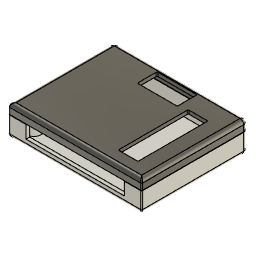
Diag_UP_PCB_v0 v13 (Autodesk Fusion 360 design; units mm, degrees)
Autodesk Fusion 360 part; units mm, degrees
(part 1 of 2)
sketch "Skizze1" plane through (0, 0, 0) normal (0, 0, 1) x (1, 0, 0)
  line L0 (32.8826, 44.1379) -> (33.5317, 44.1379)
  line L1 (32.3975, 53.0162) -> (32.2388, 53.0162)
  line L2 (32.08, 52.8575) -> (32.2388, 53.0162)
  line L3 (31.9213, 53.0162) -> (31.7625, 53.0162)
  line L4 (33.3369, 44.3976) -> (33.3369, 43.8783)
  line L5 (29.286, 48.984) -> (29.286, 48.476)
  line L6 (27.254, 48.476) -> (27.254, 48.984)
  line L7 (31.7625, 53.0162) -> (31.6038, 53.0162)
  line L8 (26.746, 51.016) -> (27.254, 51.016)
  line L9 (29.794, 48.476) -> (29.794, 48.984)
  line L10 (33.1422, 45.0467) -> (32.8826, 44.1379)
  line L11 (27.254, 48.984) -> (26.746, 48.984)
  line L12 (27.254, 51.524) -> (26.746, 51.524)
  line L13 (29.794, 48.984) -> (29.286, 48.984)
  arc A0 (34.62, 45.3962) -> (35.89, 45.3962) centre (35.255, 45.3962) ccw
  line L14 (32.334, 48.476) -> (32.334, 48.984)
  line L15 (32.715, 53.0162) -> (32.5563, 53.0162)
  line L16 (31.445, 53.0162) -> (32.08, 52.3812)
  line L17 (36.3663, 46.19) -> (35.89, 46.6662)
  line L18 (32.08, 52.6987) -> (32.3975, 53.0162)
  line L19 (31.6038, 53.0162) -> (31.445, 53.0162)
  line L20 (24.206, 51.016) -> (24.714, 51.016)
  line L21 (22.174, 51.016) -> (22.174, 51.524)
  line L22 (24.714, 48.984) -> (24.206, 48.984)
  line L23 (22.174, 48.984) -> (21.666, 48.984)
  line L24 (24.714, 48.476) -> (24.714, 48.984)
  line L25 (29.794, 51.016) -> (29.794, 51.524)
  arc A1 (18.11, 45.3962) -> (19.38, 45.3962) centre (18.745, 45.3962) ccw
  line L26 (36.3663, 53.81) -> (35.89, 53.3338)
  line L27 (31.826, 48.476) -> (32.334, 48.476)
  line L28 (24.206, 48.476) -> (24.714, 48.476)
  line L29 (26.746, 48.476) -> (27.254, 48.476)
  line L30 (21.666, 51.016) -> (22.174, 51.016)
  line L31 (32.334, 51.016) -> (32.334, 51.524)
  line L32 (27.254, 51.016) -> (27.254, 51.524)
  line L33 (31.826, 48.984) -> (31.826, 48.476)
  line L34 (21.666, 48.476) -> (22.174, 48.476)
  line L35 (31.826, 51.524) -> (31.826, 51.016)
  line L36 (26.746, 48.984) -> (26.746, 48.476)
  line L37 (21.666, 51.524) -> (21.666, 51.016)
  line L38 (29.286, 51.524) -> (29.286, 51.016)
  arc A2 (26.5238, 45.3962) -> (27.635, 45.3962) centre (27.0794, 45.3962) ccw
  line L39 (21.666, 48.984) -> (21.666, 48.476)
  line L40 (32.0956, 43.8783) -> (31.9657, 43.8783)
  line L41 (24.206, 48.984) -> (24.206, 48.476)
  line L42 (32.08, 52.3812) -> (32.715, 53.0162)
  line L43 (29.0638, 53.81) -> (36.3663, 53.81)
  line L44 (22.174, 51.524) -> (21.666, 51.524)
  arc A3 (32.0956, 43.8783) -> (32.3552, 44.1379) centre (32.0956, 44.1379) ccw
  line L45 (24.714, 51.016) -> (24.714, 51.524)
  line L46 (32.5563, 53.0162) -> (32.3975, 53.0162)
  line L47 (32.08, 52.54) -> (32.5563, 53.0162)
  line L48 (29.794, 51.524) -> (29.286, 51.524)
  line L49 (18.11, 53.3338) -> (17.6337, 53.81)
  line L50 (17.6337, 48.2537) -> (17.6337, 53.81)
  line L51 (29.286, 51.016) -> (29.794, 51.016)
  line L52 (32.334, 48.984) -> (31.826, 48.984)
  line L53 (24.206, 51.524) -> (24.206, 51.016)
  line L54 (26.746, 51.524) -> (26.746, 51.016)
  line L55 (22.174, 48.476) -> (22.174, 48.984)
  line L56 (24.714, 51.524) -> (24.206, 51.524)
  line L57 (32.3552, 45.0467) -> (32.3552, 44.1379)
  line L58 (29.286, 48.476) -> (29.794, 48.476)
  line L59 (35.4013, 18.415) -> (35.4013, 17.653)
  line L60 (40.0695, 44.5417) -> (40.3941, 44.5417)
  line L61 (39.37, 33.4963) -> (39.37, 41.1163)
  line L62 (39.6875, 41.1163) -> (39.6875, 33.4963)
  line L63 (40.0695, 43.3733) -> (40.0695, 44.5417)
  line L64 (41.5297, 44.5417) -> (41.5297, 43.3733)
  line L65 (36.83, 41.1163) -> (36.83, 33.4963)
  line L66 (41.2052, 44.2821) -> (41.5297, 44.5417)
  line L67 (40.9575, 41.1163) -> (40.9575, 41.8783)
  line L68 (42.2275, 41.1163) -> (39.6875, 41.1163)
  line L69 (36.6713, 18.415) -> (36.6713, 26.035)
  arc A4 (38.7569, 44.1649) -> (38.8543, 44.3921) centre (38.5405, 44.3921) ccw
  line L70 (40.3941, 43.8926) -> (40.0695, 43.8926)
  line L71 (34.1313, 26.035) -> (34.1313, 18.415)
  arc A5 (38.8543, 44.3921) -> (38.5622, 44.6842) centre (38.5622, 44.3921) ccw
  line L72 (37.3941, 44.0351) -> (37.0695, 44.0351)
  line L73 (39.37, 41.1163) -> (36.83, 41.1163)
  line L74 (38.1, 41.1163) -> (38.1, 41.8783)
  line L75 (36.83, 33.4963) -> (39.37, 33.4963)
  line L76 (37.0695, 44.6842) -> (37.3941, 44.6842)
  line L77 (40.9575, 33.4963) -> (40.9575, 32.7343)
  line L78 (39.6875, 33.4963) -> (42.2275, 33.4963)
  line L79 (37.0695, 43.5158) -> (37.0695, 44.6842)
  line L80 (37.7187, 43.5158) -> (37.459, 44.0351)
  line L81 (40.7187, 43.3733) -> (40.459, 43.8926)
  line L82 (42.2275, 33.4963) -> (42.2275, 41.1163)
  arc A6 (40.3941, 43.8925) -> (40.3941, 44.5417) centre (40.3941, 44.2171) ccw
  line L83 (38.2052, 43.5158) -> (38.8543, 43.5158)
  arc A7 (37.3941, 44.035) -> (37.3941, 44.6842) centre (37.3941, 44.3596) ccw
  line L84 (38.7569, 44.1649) -> (38.2052, 43.5158)
  line L85 (38.1, 33.4963) -> (38.1, 32.7343)
  line L86 (41.2052, 43.3733) -> (41.8543, 43.3733)
  arc A8 (38.5622, 44.6842) -> (38.2052, 44.4245) centre (38.5622, 44.3089) ccw
  line L87 (5.89, 0.1) -> (5.89, -1)
  line L88 (30.38, 0) -> (30.38, -1)
  line L89 (13.31, 3) -> (13.31, 2)
  line L90 (13.81, 0.1) -> (13.81, 4)
  line L91 (16.27, 3) -> (16.27, 2)
  arc A9 (28.15, 2) -> (29.15, 2) centre (28.65, 2) ccw
  arc A10 (17.27, 3) -> (16.27, 3) centre (16.77, 3) ccw
  line L92 (19, -1) -> (19, 0)
  line L93 (26.92, 0) -> (26.42, 0)
  line L94 (17.77, 0.1) -> (17.77, -1)
  line L95 (15.04, -1) -> (15.04, 0)
  line L96 (17.77, 0.1) -> (17.77, 4)
  line L97 (24.19, 3) -> (24.19, 2)
  line L98 (13.81, 0.1) -> (13.81, -1)
  arc A11 (13.31, 3) -> (12.31, 3) centre (12.81, 3) ccw
  line L99 (17.27, 3) -> (17.27, 2)
  line L100 (11.08, -1) -> (11.08, 0)
  line L101 (21.73, 0.1) -> (21.73, -1)
  line L102 (23.69, 0.1) -> (23.69, -1)
  arc A12 (17.77, 4) -> (15.77, 4) centre (16.77, 4) ccw
  line L103 (21.73, 0.1) -> (21.73, 4)
  line L104 (14.54, 0) -> (14.54, -1)
  line L105 (11.08, 0) -> (10.58, 0)
  line L106 (12.31, 3) -> (12.31, 2)
  arc A13 (13.81, 4) -> (11.81, 4) centre (12.81, 4) ccw
  arc A14 (16.27, 2) -> (17.27, 2) centre (16.77, 2) ccw
  line L107 (6.62, 0) -> (6.62, -1)
  line L108 (30.88, 0) -> (30.38, 0)
  line L109 (21.23, 3) -> (21.23, 2)
  line L110 (3.89, 0.1) -> (3.89, 4)
  arc A15 (24.19, 2) -> (25.19, 2) centre (24.69, 2) ccw
  line L111 (18.5, 0) -> (18.5, -1)
  arc A16 (25.69, 4) -> (23.69, 4) centre (24.69, 4) ccw
  line L112 (29.65, 0.1) -> (29.65, 4)
  arc A17 (21.73, 4) -> (19.73, 4) centre (20.73, 4) ccw
  line L113 (11.81, 0.1) -> (11.81, 4)
  line L114 (20.23, 3) -> (20.23, 2)
  line L115 (15.04, 0) -> (14.54, 0)
  arc A18 (12.31, 2) -> (13.31, 2) centre (12.81, 2) ccw
  arc A19 (9.35, 3) -> (8.35, 3) centre (8.85, 3) ccw
  line L116 (15.77, 0.1) -> (15.77, -1)
  line L117 (19.73, 0.1) -> (19.73, -1)
  line L118 (9.85, 0.1) -> (9.85, 4)
  arc A20 (8.35, 2) -> (9.35, 2) centre (8.85, 2) ccw
  line L119 (7.12, 0) -> (6.62, 0)
  line L120 (11.81, 0.1) -> (11.81, -1)
  line L121 (19.73, 0.1) -> (19.73, 4)
  arc A21 (21.23, 3) -> (20.23, 3) centre (20.73, 3) ccw
  line L122 (10.58, 0) -> (10.58, -1)
  arc A22 (20.23, 2) -> (21.23, 2) centre (20.73, 2) ccw
  line L123 (19, 0) -> (18.5, 0)
  line L124 (2.66, 0) -> (2.66, -1)
  line L125 (4.39, 3) -> (4.39, 2)
  line L126 (7.12, -1) -> (7.12, 0)
  line L127 (5.89, 0.1) -> (5.89, 4)
  line L128 (15.77, 0.1) -> (15.77, 4)
  line L129 (28.15, 3) -> (28.15, 2)
  line L130 (22.46, 0) -> (22.46, -1)
  arc A23 (9.85, 4) -> (7.85, 4) centre (8.85, 4) ccw
  arc A24 (5.89, 4) -> (3.89, 4) centre (4.89, 4) ccw
  line L131 (8.35, 3) -> (8.35, 2)
  line L132 (-6.03, 0) -> (-7.58, 0)
  line L133 (-0.13, -1) -> (-0.13, 0)
  line L134 (-6.03, -1.6) -> (-6.03, 0)
  line L135 (59.37, -6.8) -> (55.97, -6.8)
  line L136 (59.37, 0) -> (57.67, 0)
  line L137 (7.85, 0.1) -> (7.85, 4)
  line L138 (-6.03, -6.8) -> (-6.03, -5.2)
  line L139 (60.92, -6.8) -> (59.37, -6.8)
  line L140 (3.89, 0.1) -> (3.89, -1)
  line L141 (5.39, 3) -> (5.39, 2)
  line L142 (59.37, -6.8) -> (59.37, -5.2)
  line L143 (3.16, -1) -> (3.16, 0)
  line L144 (57.67, -2.8667) -> (57.67, 0)
  line L145 (57.67, -3.6853) -> (57.67, -3.548)
  line L146 (-4.33, 0) -> (-6.03, 0)
  line L147 (-4.33, -4.3667) -> (-4.33, -7.2333)
  line L148 (57.67, 0) -> (55.97, 0)
  line L149 (-0.83, -6.8) -> (-2.63, -6.8)
  arc A25 (4.39, 2) -> (5.39, 2) centre (4.89, 2) ccw
  line L150 (-4.33, -8.7333) -> (-4.33, -11.6)
  line L151 (7.85, 0.1) -> (7.85, -1)
  line L152 (-0.83, -11.6) -> (-0.83, -6.8)
  line L153 (55.97, -6.8) -> (54.17, -6.8)
  line L154 (53.47, -1) -> (-0.13, -1)
  line L155 (-6.03, -4.2) -> (-6.03, -2.6)
  line L156 (3.16, 0) -> (2.66, 0)
  line L157 (9.85, 0.1) -> (9.85, -1)
  line L158 (59.37, -4.2) -> (59.37, -2.6)
  line L159 (-2.63, -6.8) -> (-2.63, -5.2)
  line L160 (57.67, -7.2333) -> (57.67, -4.3667)
  line L161 (9.35, 3) -> (9.35, 2)
  line L162 (-4.33, -7.9147) -> (-4.33, -8.052)
  line L163 (55.97, 0) -> (53.47, 0)
  line L164 (-0.13, 0) -> (-2.63, 0)
  line L165 (53.47, 0) -> (53.47, -1)
  line L166 (-2.63, 0) -> (-4.33, 0)
  line L167 (60.92, 0) -> (59.37, 0)
  line L168 (-2.63, -6.8) -> (-6.03, -6.8)
  line L169 (60.92, 0) -> (60.92, -6.8)
  line L170 (57.67, -8.052) -> (57.67, -7.9147)
  line L171 (-2.63, -4.2) -> (-2.63, -2.6)
  arc A26 (5.39, 3) -> (4.39, 3) centre (4.89, 3) ccw
  line L172 (-7.58, 0) -> (-7.58, -6.8)
  line L173 (-4.33, -3.548) -> (-4.33, -3.6853)
  line L174 (52.6038, 8.38) -> (46.2537, 8.38)
  line L175 (51.5814, 0.7496) -> (52.2305, 0.7496)
  line L176 (51.3338, 9.65) -> (46.2537, 9.65)
  line L177 (54.17, -11.6) -> (-0.83, -11.6)
  line L178 (46.2537, 9.65) -> (44.825, 9.65)
  line L179 (44.825, 9.65) -> (44.6662, 9.65)
  line L180 (51.5814, 1.6583) -> (51.9059, 1.918)
  line L181 (51.3338, 14.73) -> (51.3338, 9.65)
  line L182 (51.3338, 14.73) -> (51.81, 14.73)
  line L183 (51.9059, 1.918) -> (51.9059, 0.7496)
  line L184 (51.054, 1.918) -> (51.054, 1.0092)
  line L185 (46.2537, 23.62) -> (52.6038, 23.62)
  line L186 (44.825, 8.38) -> (43.3962, 8.38)
  line L187 (44.825, 22.35) -> (46.2537, 22.35)
  line L188 (43.3962, 23.62) -> (44.825, 23.62)
  line L189 (-6.03, -6.8) -> (-7.58, -6.8)
  line L190 (54.17, -6.8) -> (54.17, -11.6)
  line L191 (50.7944, 0.7496) -> (50.6646, 0.7496)
  line L192 (51.3338, 17.27) -> (51.3338, 14.73)
  line L193 (-4.33, 0) -> (-4.33, -2.8667)
  line L194 (57.67, -11.6) -> (57.67, -8.7333)
  line L195 (-2.63, -1.6) -> (-2.63, 0)
  line L196 (51.3338, 22.35) -> (51.3338, 17.27)
  line L197 (51.81, 14.73) -> (52.6038, 14.73)
  line L198 (51.81, 9.1737) -> (51.3338, 9.65)
  line L199 (51.0162, 13.7775) -> (51.0162, 13.9362)
  line L200 (46.2537, 22.8263) -> (51.81, 22.8263)
  line L201 (46.2537, 22.8263) -> (46.2537, 23.62)
  line L202 (46.2537, 9.1737) -> (51.81, 9.1737)
  line L203 (46.2537, 22.35) -> (51.3338, 22.35)
  line L204 (44.19, 9.1737) -> (44.6662, 9.65)
  line L205 (55.97, -4.2) -> (55.97, -2.6)
  line L206 (52.6038, 23.62) -> (52.6038, 17.27)
  line L207 (52.6038, 14.73) -> (52.6038, 8.38)
  arc A27 (50.7944, 0.7496) -> (51.054, 1.0092) centre (50.7944, 1.0092) ccw
  line L208 (50.54, 13.46) -> (51.0162, 12.9837)
  line L209 (46.2537, 22.35) -> (46.2537, 22.8263)
  line L210 (44.825, 22.8263) -> (44.19, 22.8263)
  line L211 (55.97, -6.8) -> (55.97, -5.2)
  line L212 (44.825, 9.65) -> (44.825, 9.1737)
  line L213 (51.3338, 17.27) -> (51.81, 17.27)
  line L214 (50.3812, 13.46) -> (51.0162, 12.825)
  line L215 (51.81, 17.27) -> (51.81, 22.8263)
  line L216 (44.6662, 22.35) -> (44.19, 22.8263)
  line L217 (46.2537, 9.1737) -> (46.2537, 8.38)
  line L218 (44.825, 22.35) -> (44.825, 22.8263)
  line L219 (51.81, 14.73) -> (51.81, 9.1737)
  arc A28 (43.3962, 16.4763) -> (43.3962, 15.3651) centre (43.3962, 15.9207) ccw
  line L220 (51.0162, 13.9362) -> (51.0162, 14.095)
  line L221 (46.2537, 8.38) -> (44.825, 8.38)
  line L222 (44.6662, 9.65) -> (44.6662, 22.35)
  line L223 (52.6038, 17.27) -> (52.6038, 14.73)
  line L224 (44.19, 9.1737) -> (44.19, 22.8263)
  line L225 (51.81, 17.27) -> (52.6038, 17.27)
  line L226 (44.825, 9.1737) -> (44.825, 8.38)
  line L227 (44.825, 22.8263) -> (44.825, 23.62)
  line L228 (59.37, -1.6) -> (59.37, 0)
  line L229 (43.3962, 8.38) -> (43.3962, 23.62)
  line L230 (44.6662, 22.35) -> (44.825, 22.35)
  line L231 (44.19, 9.1737) -> (44.825, 9.1737)
  arc A29 (43.3962, 10.92) -> (43.3962, 9.65) centre (43.3962, 10.285) ccw
  line L232 (51.0162, 12.825) -> (51.0162, 12.9837)
  line L233 (51.0162, 14.095) -> (50.3812, 13.46)
  line L234 (46.2537, 9.65) -> (46.2537, 9.1737)
  line L235 (44.825, 23.62) -> (46.2537, 23.62)
  line L236 (51.3338, 22.35) -> (51.81, 22.8263)
  arc A30 (43.3962, 22.35) -> (43.3962, 21.08) centre (43.3962, 21.715) ccw
  line L237 (51.0162, 13.9362) -> (50.54, 13.46)
  line L238 (55.97, -1.6) -> (55.97, 0)
  line L239 (43.3962, 24.84) -> (43.3962, 45.16)
  line L240 (52.6038, 32.9362) -> (52.6038, 24.84)
  line L241 (44.825, 25.6337) -> (44.825, 24.84)
  line L242 (49.524, 13.206) -> (49.524, 13.714)
  line L243 (46.2537, 26.11) -> (46.2537, 25.6337)
  line L244 (46.2537, 43.89) -> (51.3338, 43.89)
  line L245 (42.6867, 14.7564) -> (42.6867, 15.4055)
  line L246 (49.016, 18.794) -> (49.016, 18.286)
  line L247 (51.3338, 43.89) -> (51.3338, 37.0638)
  line L248 (49.524, 15.746) -> (49.524, 16.254)
  line L249 (46.984, 15.746) -> (46.984, 16.254)
  line L250 (46.476, 18.794) -> (46.476, 18.286)
  line L251 (49.524, 13.714) -> (49.016, 13.714)
  line L252 (46.2537, 45.16) -> (52.6038, 45.16)
  line L253 (46.984, 13.206) -> (46.984, 13.714)
  line L254 (51.0162, 13.6187) -> (50.8575, 13.46)
  arc A31 (41.5183, 15.1134) -> (41.778, 14.7564) centre (41.8936, 15.1134) ccw
  line L255 (51.0162, 13.3012) -> (51.0162, 13.6187)
  line L256 (49.016, 18.286) -> (49.524, 18.286)
  line L257 (42.6867, 13.9694) -> (42.6867, 13.8396)
  line L258 (46.984, 18.794) -> (46.476, 18.794)
  line L259 (46.476, 13.714) -> (46.476, 13.206)
  line L260 (46.476, 15.746) -> (46.984, 15.746)
  line L261 (49.524, 18.794) -> (49.016, 18.794)
  arc A32 (42.6867, 13.9694) -> (42.4271, 14.229) centre (42.4271, 13.9694) ccw
  line L262 (46.2537, 26.11) -> (44.825, 26.11)
  line L263 (49.524, 16.254) -> (49.016, 16.254)
  arc A33 (41.8104, 15.4055) -> (41.5183, 15.1134) centre (41.8104, 15.1134) ccw
  line L264 (51.3338, 37.0638) -> (51.81, 37.0638)
  line L265 (44.825, 45.16) -> (46.2537, 45.16)
  line L266 (49.016, 13.206) -> (49.524, 13.206)
  line L267 (46.984, 13.714) -> (46.476, 13.714)
  line L268 (46.984, 18.286) -> (46.984, 18.794)
  line L269 (52.6038, 37.0638) -> (52.6038, 32.9362)
  line L270 (44.825, 44.3663) -> (44.825, 45.16)
  line L271 (44.825, 26.11) -> (44.825, 25.6337)
  line L272 (44.6662, 26.11) -> (44.6662, 43.89)
  line L273 (50.6987, 13.46) -> (51.0162, 13.1425)
  line L274 (46.476, 16.254) -> (46.476, 15.746)
  line L275 (49.016, 15.746) -> (49.524, 15.746)
  arc A34 (42.0376, 15.3081) -> (41.8104, 15.4055) centre (41.8104, 15.0918) ccw
  line L276 (41.5183, 14.2291) -> (42.4271, 14.2291)
  line L277 (51.0162, 13.1425) -> (51.0162, 13.3012)
  line L278 (46.984, 16.254) -> (46.476, 16.254)
  line L279 (51.0162, 12.9837) -> (51.0162, 13.1425)
  line L280 (51.0162, 13.7775) -> (50.6987, 13.46)
  line L281 (46.476, 18.286) -> (46.984, 18.286)
  line L282 (50.8575, 13.46) -> (51.0162, 13.3012)
  line L283 (49.524, 18.286) -> (49.524, 18.794)
  line L284 (46.476, 13.206) -> (46.984, 13.206)
  line L285 (49.016, 13.714) -> (49.016, 13.206)
  line L286 (51.3338, 26.11) -> (46.2537, 26.11)
  line L287 (49.016, 16.254) -> (49.016, 15.746)
  line L288 (44.825, 43.89) -> (44.825, 44.3663)
  line L289 (51.0162, 13.6187) -> (51.0162, 13.7775)
  line L290 (51.81, 32.9362) -> (51.81, 25.6337)
  line L291 (51.0162, 30.0787) -> (50.8575, 29.92)
  line L292 (51.0162, 30.3962) -> (50.54, 29.92)
  line L293 (51.81, 32.9362) -> (52.6038, 32.9362)
  line L294 (45.3675, 6.9448) -> (44.8708, 7.2157)
  line L295 (46.984, 32.206) -> (46.984, 32.714)
  line L296 (44.825, 44.3663) -> (44.19, 44.3663)
  line L297 (51.3338, 32.9362) -> (51.81, 32.9362)
  line L298 (51.3338, 37.0638) -> (51.3338, 32.9362)
  line L299 (51.0162, 29.6025) -> (51.0162, 29.7612)
  line L300 (44.6662, 43.89) -> (44.825, 43.89)
  line L301 (46.2537, 43.89) -> (46.2537, 44.3663)
  line L302 (52.4567, 6.2675) -> (51.7342, 6.2675)
  line L303 (45.411, 47.263) -> (46.3142, 47.263)
  line L304 (44.19, 25.6337) -> (44.825, 25.6337)
  line L305 (46.9312, 45.6375) -> (46.9312, 47.263)
  line L306 (51.0162, 29.285) -> (51.0162, 29.4437)
  line L307 (44.6662, 43.89) -> (44.19, 44.3663)
  line L308 (44.825, 26.11) -> (44.6662, 26.11)
  line L309 (52.6038, 24.84) -> (46.2537, 24.84)
  line L310 (51.0162, 30.0787) -> (51.0162, 30.2375)
  arc A35 (43.3962, 27.38) -> (43.3962, 26.11) centre (43.3962, 26.745) ccw
  arc A36 (46.9167, 7.7575) -> (46.5103, 7.893) centre (46.5103, 7.2157) ccw
  line L311 (51.81, 37.0638) -> (52.6038, 37.0638)
  line L312 (51.81, 25.6337) -> (51.3338, 26.11)
  line L313 (46.2537, 25.6337) -> (51.81, 25.6337)
  line L314 (50.3812, 29.92) -> (51.0162, 29.285)
  line L315 (46.2537, 24.84) -> (44.825, 24.84)
  line L316 (52.6038, 45.16) -> (52.6038, 37.0638)
  line L317 (51.0162, 30.555) -> (50.3812, 29.92)
  line L318 (50.54, 29.92) -> (51.0162, 29.4437)
  line L319 (51.0162, 30.2375) -> (51.0162, 30.3962)
  line L320 (50.6987, 29.92) -> (51.0162, 29.6025)
  arc A37 (47.0071, 6.6287) -> (46.8265, 6.9448) centre (46.6402, 6.6287) ccw
  line L321 (44.19, 25.6337) -> (44.6662, 26.11)
  line L322 (46.2537, 44.3663) -> (51.81, 44.3663)
  arc A38 (43.3962, 35.4763) -> (43.3962, 34.3651) centre (43.3962, 34.9207) ccw
  arc A39 (45.0514, 7.893) -> (44.6902, 7.5318) centre (45.0514, 7.5318) ccw
  line L323 (43.3962, 45.16) -> (44.825, 45.16)
  line L324 (51.0162, 29.4437) -> (51.0162, 29.6025)
  line L325 (46.2537, 25.6337) -> (46.2537, 24.84)
  line L326 (51.0162, 30.3962) -> (51.0162, 30.555)
  line L327 (51.7342, 6.2675) -> (51.7342, 7.8931)
  arc A40 (45.4578, 7.7575) -> (45.0514, 7.893) centre (45.0514, 7.2157) ccw
  arc A41 (46.104, 6.4933) -> (46.6458, 6.2675) centre (46.6458, 7.0306) ccw
  line L328 (49.317, 6.2675) -> (49.317, 7.8931)
  line L329 (42.0376, 15.3081) -> (42.6867, 14.7564)
  line L330 (51.3338, 32.9362) -> (51.3338, 26.11)
  line L331 (50.8575, 29.92) -> (51.0162, 29.7612)
  line L332 (51.0162, 29.7612) -> (51.0162, 30.0787)
  line L333 (45.8626, 45.6375) -> (45.8626, 47.263)
  line L334 (44.825, 43.89) -> (46.2537, 43.89)
  arc A42 (43.3962, 43.89) -> (43.3962, 42.62) centre (43.3962, 43.255) ccw
  line L335 (47.67, 7.8931) -> (48.3925, 7.8931)
  line L336 (44.825, 24.84) -> (43.3962, 24.84)
  line L337 (50.6717, 6.2675) -> (50.6717, 7.8931)
  line L338 (46.2537, 44.3663) -> (46.2537, 45.16)
  line L339 (51.81, 37.0638) -> (51.81, 44.3663)
  line L340 (50.2202, 7.8931) -> (51.1233, 7.8931)
  line L341 (51.0162, 30.2375) -> (50.6987, 29.92)
  line L342 (51.3338, 43.89) -> (51.81, 44.3663)
  line L343 (44.19, 25.6337) -> (44.19, 44.3663)
  arc A43 (45.5481, 6.6287) -> (45.3675, 6.9448) centre (45.1812, 6.6287) ccw
  line L344 (48.3925, 6.2675) -> (47.67, 6.2675)
  arc A44 (46.6458, 6.2675) -> (47.007, 6.6287) centre (46.6458, 6.6287) ccw
  line L345 (37.827, 47.1573) -> (37.827, 48.0604)
  line L346 (48.8655, 7.8931) -> (49.7686, 7.8931)
  arc A45 (44.6902, 7.5318) -> (44.8708, 7.2157) centre (45.0571, 7.5318) ccw
  arc A46 (5.1626, 14.8153) -> (4.711, 15.2669) centre (4.711, 14.8153) ccw
  line L347 (0, 1) -> (0, 54)
  line L348 (3.9885, 15.2668) -> (4.711, 15.2668)
  arc A47 (47.3828, 46.3599) -> (47.3828, 47.2631) centre (47.3828, 46.8115) ccw
  line L349 (44.2087, 45.9987) -> (44.2087, 46.9018)
  line L350 (47.8343, 45.6375) -> (47.4731, 46.3599)
  line L351 (49.8017, 46.7212) -> (50.8854, 46.7212)
  arc A48 (52, 0) -> (53, 1) centre (52, 1) ccw
  arc A49 (0, 1) -> (1, 0) centre (1, 1) ccw
  line L352 (47.67, 7.1706) -> (48.2119, 7.1706)
  arc A50 (44.2087, 45.9987) -> (44.5699, 45.6375) centre (44.5699, 45.9987) ccw
  line L353 (47.67, 6.2675) -> (47.67, 7.8931)
  line L354 (39.4526, 46.6774) -> (39.4526, 46.3162)
  arc A51 (39.0913, 45.955) -> (39.4525, 46.3162) centre (39.0913, 46.3162) ccw
  line L355 (46.9312, 47.263) -> (47.3828, 47.263)
  arc A52 (53, 54) -> (52, 55) centre (52, 54) ccw
  line L356 (39.4526, 48.6775) -> (37.827, 48.6775)
  arc A53 (1, 55) -> (0, 54) centre (1, 54) ccw
  line L357 (3.537, 14.3637) -> (3.537, 14.8153)
  arc A54 (4.6207, 21.1545) -> (4.2595, 20.7933) centre (4.6207, 20.7933) ccw
  line L358 (48.5403, 45.6375) -> (49.2628, 45.6375)
  line L359 (37.827, 46.3162) -> (37.827, 46.6774)
  line L360 (50.6145, 45.6375) -> (50.6145, 47.263)
  line L361 (53, 1) -> (53, 54)
  line L362 (4.5304, 17.3054) -> (4.5304, 16.899)
  line L363 (46.8264, 6.9448) -> (46.3297, 7.2157)
  arc A55 (37.8269, 46.3162) -> (38.1882, 45.9549) centre (38.1882, 46.3162) ccw
  arc A56 (46.5103, 7.893) -> (46.1491, 7.5318) centre (46.5103, 7.5318) ccw
  arc A57 (44.5699, 47.263) -> (44.2087, 46.9018) centre (44.5699, 46.9018) ccw
  arc A58 (46.1491, 7.5318) -> (46.3297, 7.2157) centre (46.516, 7.5318) ccw
  line L364 (48.5403, 47.263) -> (48.5403, 45.6375)
  line L365 (51.7342, 7.8931) -> (52.4567, 7.8931)
  line L366 (44.5699, 47.263) -> (44.9312, 47.263)
  line L367 (51.5072, 46.9018) -> (51.9588, 47.263)
  line L368 (51.9588, 47.263) -> (51.9588, 45.6375)
  line L369 (50.0726, 45.6375) -> (50.0726, 47.263)
  line L370 (39.4526, 47.6088) -> (37.827, 47.6088)
  line L371 (51.5072, 45.6375) -> (52.4103, 45.6375)
  line L372 (51.7342, 7.1706) -> (52.276, 7.1706)
  line L373 (44.9312, 45.6375) -> (44.5699, 45.6375)
  line L374 (47.3828, 46.3599) -> (46.9312, 46.3599)
  line L375 (1, 0) -> (52, 0)
  line L376 (5.1626, 14.3637) -> (3.537, 14.3637)
  line L377 (49.8017, 46.1793) -> (50.8854, 46.1793)
  line L378 (39.0913, 45.955) -> (38.1882, 45.955)
  arc A59 (3.9885, 15.2669) -> (3.5369, 14.8153) centre (3.9885, 14.8153) ccw
  line L379 (52, 55) -> (1, 55)
  line L380 (4.0788, 17.0345) -> (4.0788, 16.6733)
  line L381 (4.2594, 20.7933) -> (4.2594, 20.2515)
  line L382 (4.2594, 20.2515) -> (3.537, 20.2515)
  line L383 (4.711, 32.7043) -> (4.5304, 32.2528)
  arc A60 (4.711, 30.5159) -> (4.711, 31.4191) centre (4.711, 30.9675) ccw
  line L384 (4.0788, 18.2607) -> (4.0788, 18.7122)
  arc A61 (4.3498, 17.3054) -> (4.0789, 17.0345) centre (4.3498, 17.0345) ccw
  arc A62 (4.5304, 16.899) -> (5.1626, 16.899) centre (4.8465, 16.899) ccw
  line L385 (4.711, 31.4191) -> (3.537, 31.4191)
  arc A63 (3.7628, 28.2026) -> (4.3498, 28.0671) centre (4.3498, 29.4067) ccw
  line L386 (5.1626, 16.899) -> (5.1626, 17.3054)
  arc A64 (4.3498, 28.9701) -> (3.7628, 28.8346) centre (4.3498, 27.6305) ccw
  line L387 (5.1626, 17.3054) -> (4.3498, 17.3054)
  arc A65 (4.0789, 18.2607) -> (4.3498, 17.9898) centre (4.3498, 18.2607) ccw
  arc A66 (5.0722, 32.1173) -> (5.1625, 32.614) centre (3.6311, 32.6359) ccw
  line L388 (3.6273, 15.9164) -> (3.537, 15.9164)
  line L389 (3.537, 15.9164) -> (3.537, 16.0067)
  arc A67 (3.537, 27.0007) -> (3.8982, 26.504) centre (4.0591, 27.0007) ccw
  arc A68 (3.8982, 21.9049) -> (3.8982, 22.6273) centre (3.8982, 22.2661) ccw
  line L390 (4.2594, 25.7085) -> (5.1626, 24.9408)
  arc A69 (4.9368, 28.8346) -> (4.3498, 28.9701) centre (4.3498, 27.6305) ccw
  line L391 (5.1626, 15.9615) -> (4.0788, 15.9615)
  arc A70 (4.711, 21.8145) -> (4.711, 22.7177) centre (4.711, 22.2661) ccw
  line L392 (4.8013, 21.1546) -> (4.6207, 21.1546)
  arc A71 (4.711, 23.3777) -> (4.711, 24.2809) centre (4.711, 23.8293) ccw
  line L393 (5.1626, 20.2515) -> (5.1626, 20.7933)
  arc A72 (3.537, 25.4375) -> (3.8982, 24.9408) centre (4.0591, 25.4375) ccw
  arc A73 (4.2595, 27.2715) -> (3.9434, 27.407) centre (3.9434, 26.9705) ccw
  line L394 (3.537, 20.2515) -> (3.537, 21.1546)
  line L395 (3.537, 16.0067) -> (3.6273, 16.0067)
  arc A74 (4.8916, 17.9898) -> (5.1625, 18.2607) centre (4.8916, 18.2607) ccw
  line L396 (4.8916, 17.9898) -> (4.3498, 17.9898)
  arc A75 (4.711, 22.7177) -> (4.711, 21.8145) centre (4.711, 22.2661) ccw
  arc A76 (4.6207, 24.2808) -> (4.2595, 23.9196) centre (4.6207, 23.9196) ccw
  line L397 (4.2594, 23.3777) -> (4.2594, 23.9196)
  arc A77 (3.9434, 25.8439) -> (3.537, 25.4375) centre (3.9434, 25.4375) ccw
  line L398 (4.2594, 27.2716) -> (5.1626, 26.5039)
  arc A78 (5.1625, 20.7933) -> (4.8013, 21.1545) centre (4.8013, 20.7933) ccw
  arc A79 (5.7044, 18.4413) -> (5.4335, 18.7122) centre (5.4335, 18.4413) ccw
  arc A80 (3.5369, 24.1002) -> (4.2594, 23.3777) centre (4.2594, 24.1002) ccw
  arc A81 (3.7627, 28.8347) -> (3.5369, 28.5186) centre (3.8711, 28.5186) ccw
  arc A82 (4.9368, 28.2025) -> (5.1626, 28.5186) centre (4.8284, 28.5186) ccw
  arc A83 (4.0788, 32.343) -> (4.5304, 32.2527) centre (4.313, 32.3397) ccw
  arc A84 (3.9434, 27.4071) -> (3.537, 27.0007) centre (3.9434, 27.0007) ccw
  arc A85 (5.1626, 32.614) -> (4.711, 32.7043) centre (4.9284, 32.6173) ccw
  line L399 (4.0788, 18.7122) -> (5.4335, 18.7122)
  arc A86 (4.1691, 32.7495) -> (4.0788, 32.343) centre (5.1043, 32.3284) ccw
  arc A87 (3.8982, 22.6273) -> (3.8982, 21.9049) centre (3.8982, 22.2661) ccw
  arc A88 (4.2595, 25.7084) -> (3.9434, 25.8439) centre (3.9434, 25.4074) ccw
  line L400 (5.1626, 18.7122) -> (5.1626, 18.2607)
  line L401 (5.7044, 18.4413) -> (5.7044, 18.0801)
  line L402 (4.6207, 24.2808) -> (4.711, 24.2808)
  line L403 (4.8013, 28.1574) -> (3.8982, 28.8799)
  line L404 (5.1626, 14.8153) -> (5.1626, 14.3637)
  line L405 (3.6273, 16.0067) -> (3.6273, 15.9164)
  line L406 (5.1626, 26.5039) -> (5.1626, 27.4071)
  line L407 (4.711, 23.3777) -> (4.2594, 23.3777)
  line L408 (50.68, -1) -> (50.68, 0)
  line L409 (38.8, 0) -> (38.3, 0)
  line L410 (46.72, 0) -> (46.22, 0)
  line L411 (47.45, 0.1) -> (47.45, -1)
  line L412 (32.11, 3) -> (32.11, 2)
  arc A89 (33.11, 3) -> (32.11, 3) centre (32.61, 3) ccw
  line L413 (37.07, 3) -> (37.07, 2)
  line L414 (14.0018, 20.9804) -> (14.6368, 20.4406)
  arc A90 (40.03, 2) -> (41.03, 2) centre (40.53, 2) ccw
  arc A91 (41.53, 4) -> (39.53, 4) centre (40.53, 4) ccw
  arc A92 (33.61, 4) -> (31.61, 4) centre (32.61, 4) ccw
  line L415 (41.53, 0.1) -> (41.53, -1)
  line L416 (40.03, 3) -> (40.03, 2)
  line L417 (42.26, 0) -> (42.26, -1)
  arc A93 (36.07, 2) -> (37.07, 2) centre (36.57, 2) ccw
  line L418 (50.18, 0) -> (50.18, -1)
  line L419 (41.53, 0.1) -> (41.53, 4)
  line L420 (35.57, 0.1) -> (35.57, -1)
  line L421 (38.8, -1) -> (38.8, 0)
  line L422 (30.88, -1) -> (30.88, 0)
  line L423 (26.42, 0) -> (26.42, -1)
  line L424 (36.07, 3) -> (36.07, 2)
  line L425 (39.53, 0.1) -> (39.53, -1)
  line L426 (25.69, 0.1) -> (25.69, 4)
  line L427 (26.92, -1) -> (26.92, 0)
  line L428 (39.53, 0.1) -> (39.53, 4)
  line L429 (29.15, 3) -> (29.15, 2)
  line L430 (29.65, 0.1) -> (29.65, -1)
  line L431 (34.84, -1) -> (34.84, 0)
  line L432 (23.69, 0.1) -> (23.69, 4)
  line L433 (33.11, 3) -> (33.11, 2)
  arc A94 (29.65, 4) -> (27.65, 4) centre (28.65, 4) ccw
  line L434 (46.22, 0) -> (46.22, -1)
  arc A95 (37.57, 4) -> (35.57, 4) centre (36.57, 4) ccw
  line L435 (47.45, 0.1) -> (47.45, 4)
  arc A96 (49.45, 4) -> (47.45, 4) centre (48.45, 4) ccw
  line L436 (44.99, 3) -> (44.99, 2)
  arc A97 (37.07, 3) -> (36.07, 3) centre (36.57, 3) ccw
  arc A98 (41.03, 3) -> (40.03, 3) centre (40.53, 3) ccw
  line L437 (38.3, 0) -> (38.3, -1)
  line L438 (25.19, 3) -> (25.19, 2)
  line L439 (43.49, 0.1) -> (43.49, -1)
  arc A99 (45.49, 4) -> (43.49, 4) centre (44.49, 4) ccw
  arc A100 (29.15, 3) -> (28.15, 3) centre (28.65, 3) ccw
  line L440 (27.65, 0.1) -> (27.65, 4)
  line L441 (27.65, 0.1) -> (27.65, -1)
  line L442 (22.96, -1) -> (22.96, 0)
  line L443 (25.69, 0.1) -> (25.69, -1)
  line L444 (31.61, 0.1) -> (31.61, 4)
  line L445 (22.96, 0) -> (22.46, 0)
  line L446 (31.61, 0.1) -> (31.61, -1)
  arc A101 (25.19, 3) -> (24.19, 3) centre (24.69, 3) ccw
  arc A102 (32.11, 2) -> (33.11, 2) centre (32.61, 2) ccw
  line L447 (33.61, 0.1) -> (33.61, -1)
  line L448 (34.34, 0) -> (34.34, -1)
  line L449 (35.57, 0.1) -> (35.57, 4)
  line L450 (37.57, 0.1) -> (37.57, -1)
  line L451 (37.57, 0.1) -> (37.57, 4)
  line L452 (41.03, 3) -> (41.03, 2)
  line L453 (34.84, 0) -> (34.34, 0)
  line L454 (33.61, 0.1) -> (33.61, 4)
  line L455 (46.476, 29.666) -> (46.984, 29.666)
  line L456 (46.984, 30.174) -> (46.476, 30.174)
  line L457 (49.016, 29.666) -> (49.524, 29.666)
  line L458 (49.524, 29.666) -> (49.524, 30.174)
  line L459 (46.476, 32.714) -> (46.476, 32.206)
  line L460 (49.016, 30.174) -> (49.016, 29.666)
  line L461 (37.827, 48.6775) -> (37.827, 49.129)
  line L462 (39.4526, 51.8189) -> (37.827, 51.8189)
  line L463 (38.9107, 51.5479) -> (38.9107, 52.6317)
  line L464 (46.984, 32.714) -> (46.476, 32.714)
  line L465 (46.476, 30.174) -> (46.476, 29.666)
  line L466 (38.7301, 49.129) -> (38.7301, 48.6775)
  line L467 (38.5494, 54.0211) -> (39.4526, 53.2535)
  arc A103 (37.827, 53.7502) -> (38.1882, 53.2535) centre (38.3491, 53.7502) ccw
  arc A104 (38.7301, 49.129) -> (37.8269, 49.129) centre (38.2785, 49.129) ccw
  line L468 (46.984, 29.666) -> (46.984, 30.174)
  line L469 (49.524, 30.174) -> (49.016, 30.174)
  line L470 (38.3688, 51.5479) -> (38.3688, 52.6317)
  line L471 (7.7569, 42.7687) -> (7.3674, 42.7687)
  line L472 (7.3674, 42.7687) -> (7.3674, 43.288)
  line L473 (2.9238, 3.1393) -> (2.9238, 4.0424)
  line L474 (6.7067, 34.873) -> (7.0962, 34.873)
  line L475 (8.3154, 33.7046) -> (8.3154, 34.873)
  arc A105 (9.5346, 34.5484) -> (9.21, 34.873) centre (9.21, 34.5484) ccw
  arc A106 (7.7569, 42.1196) -> (8.0165, 42.3792) centre (7.7569, 42.3792) ccw
  arc A107 (9.21, 33.7045) -> (9.5346, 34.0291) centre (9.21, 34.0291) ccw
  line L476 (8.8854, 34.873) -> (9.21, 34.873)
  line L477 (37.827, 50.2865) -> (39.4526, 50.2865)
  line L478 (2.9238, 1.5762) -> (2.9238, 2.4793)
  line L479 (39.4526, 52.3607) -> (37.827, 52.3607)
  line L480 (7.3674, 43.288) -> (8.0165, 43.288)
  line L481 (9.5346, 34.5484) -> (9.5346, 34.0291)
  line L482 (9.21, 33.7046) -> (8.8854, 33.7046)
  line L483 (7.6662, 34.873) -> (8.3154, 33.7046)
  line L484 (2.0207, 3.907) -> (2.9238, 3.1393)
  line L485 (39.4526, 49.5806) -> (38.7301, 49.2193)
  line L486 (50.2982, 3.4803) -> (51.9238, 3.4803)
  line L487 (6.447, 33.9642) -> (6.447, 34.6133)
  line L488 (7.6662, 33.7046) -> (7.6662, 34.873)
  arc A108 (2.0207, 3.9069) -> (1.7046, 4.0424) centre (1.7046, 3.6059) ccw
  line L489 (8.835, 42.1196) -> (9.2244, 43.288)
  arc A109 (38.2334, 54.1566) -> (37.827, 53.7502) centre (38.2334, 53.7502) ccw
  arc A110 (38.5495, 54.0211) -> (38.2334, 54.1566) centre (38.2334, 53.7201) ccw
  line L490 (39.4526, 53.2535) -> (39.4526, 54.1566)
  line L491 (1.2982, 2.0278) -> (2.9238, 2.0278)
  line L492 (7.3674, 42.1196) -> (7.7569, 42.1196)
  line L493 (50.6594, 3.0287) -> (50.2982, 3.4803)
  line L494 (51.9238, 3.0287) -> (51.9238, 3.9318)
  line L495 (6.0833, 42.5739) -> (6.8622, 42.5739)
  line L496 (39.4526, 50.2865) -> (39.4526, 51.009)
  line L497 (1.6594, 1.5762) -> (1.2982, 2.0278)
  line L498 (7.0962, 33.7046) -> (6.7067, 33.7046)
  line L499 (8.4455, 43.288) -> (8.835, 42.1196)
  line L500 (6.4728, 42.1845) -> (6.4728, 42.9634)
  arc A111 (1.7046, 4.0424) -> (1.2982, 3.636) centre (1.7046, 3.636) ccw
  line L501 (7.7337, 40.2146) -> (7.474, 40.7338)
  line L502 (8.8854, 33.7046) -> (8.8854, 34.873)
  line L503 (7.0962, 34.3537) -> (7.0962, 33.7046)
  line L504 (8.0165, 42.3792) -> (8.0165, 42.509)
  line L505 (6.3429, 41.383) -> (6.6026, 41.383)
  line L506 (35.7505, 35.1917) -> (36.14, 34.0233)
  arc A112 (35.0619, 34.0233) -> (35.3215, 34.2829) centre (35.0619, 34.2829) ccw
  line L507 (7.0846, 41.383) -> (7.4091, 41.383)
  arc A113 (8.0165, 42.509) -> (7.7569, 42.7686) centre (7.7569, 42.509) ccw
  arc A114 (9.8599, 41.0909) -> (9.5678, 41.383) centre (9.5678, 41.0909) ccw
  line L508 (34.6724, 35.1917) -> (35.3215, 35.1917)
  line L509 (33.9076, 32.1183) -> (33.6479, 32.1183)
  line L510 (7.4091, 40.7338) -> (7.0846, 40.7338)
  line L511 (34.6724, 34.6724) -> (34.6724, 35.1917)
  line L512 (6.6026, 40.2146) -> (6.3429, 40.2146)
  arc A115 (6.3429, 41.3829) -> (6.0833, 41.1233) centre (6.3429, 41.1233) ccw
  arc A116 (1.2982, 3.636) -> (1.6594, 3.1393) centre (1.8203, 3.636) ccw
  arc A117 (6.4471, 33.9642) -> (6.7067, 33.7046) centre (6.7067, 33.9642) ccw
  arc A118 (9.5678, 41.383) -> (9.2108, 41.1233) centre (9.5678, 41.0077) ccw
  arc A119 (35.3215, 34.4128) -> (35.0619, 34.6724) centre (35.0619, 34.4128) ccw
  line L513 (9.2108, 40.2146) -> (9.8599, 40.2146)
  line L514 (35.3215, 34.2829) -> (35.3215, 34.4128)
  line L515 (33.7778, 34.0882) -> (33.7778, 34.8671)
  line L516 (8.4686, 40.2146) -> (8.4686, 41.383)
  line L517 (35.0619, 34.6724) -> (34.6724, 34.6724)
  arc A120 (6.7067, 34.8729) -> (6.4471, 34.6133) centre (6.7067, 34.6133) ccw
  line L518 (36.14, 34.0233) -> (36.5294, 35.1917)
  arc A121 (7.4091, 40.7338) -> (7.4091, 41.383) centre (7.4091, 41.0584) ccw
  line L519 (33.3883, 34.4777) -> (34.1672, 34.4777)
  arc A122 (33.3883, 32.3779) -> (33.6479, 32.1183) centre (33.6479, 32.3779) ccw
  line L520 (8.144, 41.383) -> (8.7931, 41.383)
  line L521 (6.9014, 34.3537) -> (7.0962, 34.3537)
  arc A123 (6.0833, 40.4742) -> (6.3429, 40.2146) centre (6.3429, 40.4742) ccw
  line L522 (7.0846, 40.2146) -> (7.0846, 41.383)
  line L523 (34.6724, 34.0233) -> (35.0619, 34.0233)
  arc A124 (12.078, 26.2149) -> (11.4288, 26.2149) centre (11.7534, 26.2149) ccw
  line L524 (12.078, 36.4476) -> (12.078, 36.1879)
  arc A125 (33.6479, 33.2867) -> (33.3883, 33.0271) centre (33.6479, 33.0271) ccw
  line L525 (14.7637, 26.8288) -> (12.2238, 26.8288)
  circle A126 centre (4, 51) radius 3.1
  arc A127 (39.5258, 11.5893) -> (39.7854, 11.8489) centre (39.5258, 11.8489) ccw
  line L526 (39.9312, 8.3) -> (42.4713, 8.3)
  line L527 (32.3533, 38.481) -> (15.5893, 38.481)
  arc A128 (11.8183, 24.9346) -> (12.0779, 25.1942) centre (11.8183, 25.1942) ccw
  arc A129 (10.9095, 37.2411) -> (11.1692, 36.8841) centre (11.2848, 37.2411) ccw
  line L528 (11.4288, 37.4359) -> (12.078, 36.8841)
  arc A130 (10.9096, 25.1942) -> (11.1692, 24.9346) centre (11.1692, 25.1942) ccw
  line L529 (10.9096, 36.1879) -> (10.9096, 36.4476)
  line L530 (12.078, 25.8904) -> (12.078, 26.2149)
  line L531 (39.5258, 11.5893) -> (38.8767, 11.5893)
  line L532 (36.5158, 32.1183) -> (37.1649, 32.1183)
  arc A131 (34.7141, 32.6375) -> (34.7141, 33.2867) centre (34.7141, 32.9621) ccw
  line L533 (14.7637, 40.3225) -> (14.7637, 35.2425)
  line L534 (33.3883, 32.3779) -> (33.3883, 33.0271)
  line L535 (34.7141, 32.6376) -> (34.3896, 32.6376)
  line L536 (39.7855, 12.5451) -> (39.7855, 13.1942)
  line L537 (33.6479, 33.2867) -> (33.9076, 33.2867)
  line L538 (12.2238, 21.7488) -> (14.7637, 21.7488)
  line L539 (35.7736, 32.1183) -> (35.7736, 33.2867)
  line L540 (38.8767, 12.5451) -> (38.617, 12.8696)
  line L541 (39.9312, 8.3) -> (39.9312, 13.38)
  line L542 (12.078, 36.8841) -> (12.078, 37.5332)
  line L543 (11.8183, 24.9346) -> (11.1692, 24.9346)
  circle A132 centre (4, 51) radius 1.5875
  arc A133 (11.2017, 37.5332) -> (10.9096, 37.2411) centre (11.2017, 37.2411) ccw
  arc A134 (11.4288, 26.2798) -> (10.9096, 26.2798) centre (11.1692, 26.2798) ccw
  line L544 (10.9096, 25.1942) -> (10.9096, 25.4538)
  circle A135 centre (49, 51) radius 1.5875
  circle A136 centre (49, 51) radius 3.1
  arc A137 (38.6171, 11.8489) -> (38.8767, 11.5893) centre (38.8767, 11.8489) ccw
  line L545 (14.7637, 26.8288) -> (14.7637, 21.7488)
  arc A138 (9.7626, 40.8637) -> (9.86, 41.0909) centre (9.5462, 41.0909) ccw
  line L546 (42.4713, 13.38) -> (42.4713, 8.3)
  line L547 (38.617, 12.8696) -> (39.7855, 12.8696)
  line L548 (12.2238, 21.7488) -> (12.2238, 26.8288)
  line L549 (9.7626, 40.8637) -> (9.2108, 40.2146)
  line L550 (6.0833, 40.4742) -> (6.0833, 41.1233)
  line L551 (39.7855, 12.1086) -> (39.7855, 11.8489)
  line L552 (36.8404, 33.2867) -> (36.8404, 32.1183)
  line L553 (38.617, 11.8489) -> (38.617, 12.1086)
  line L554 (12.2238, 35.2425) -> (14.7637, 35.2425)
  line L555 (42.4713, 13.38) -> (39.9312, 13.38)
  line L556 (34.3896, 33.2867) -> (34.7141, 33.2867)
  line L557 (35.449, 33.2867) -> (36.0981, 33.2867)
  line L558 (12.2238, 35.2425) -> (12.2238, 40.3225)
  line L559 (35.0387, 32.1183) -> (34.779, 32.6376)
  arc A139 (11.4289, 37.4358) -> (11.2017, 37.5332) centre (11.2017, 37.2195) ccw
  line L560 (34.3896, 32.1183) -> (34.3896, 33.2867)
  line L561 (14.7637, 40.3225) -> (12.2238, 40.3225)
  arc A140 (10.9096, 36.188) -> (11.1692, 35.9284) centre (11.1692, 36.188) ccw
  line L562 (36.5158, 33.0271) -> (36.8404, 33.2867)
  line L563 (13.4938, 19.7384) -> (13.4938, 19.9924)
  line L564 (13.4938, 34.5694) -> (14.6368, 34.5694)
  line L565 (13.4938, 32.5755) -> (13.4938, 32.8295)
  arc A141 (14.3828, 33.2957) -> (14.6368, 33.5497) centre (14.3828, 33.5497) ccw
  line L566 (14.3828, 33.2957) -> (13.7477, 33.2957)
  line L567 (45.49, 0.1) -> (45.49, -1)
  arc A142 (15.5893, 34.544) -> (15.5893, 36.576) centre (15.5893, 35.56) ccw
  line L568 (15.5893, 38.481) -> (15.5893, 36.576)
  line L569 (43.99, 3) -> (43.99, 2)
  line L570 (15.5893, 32.639) -> (15.5893, 34.544)
  line L571 (42.76, -1) -> (42.76, 0)
  line L572 (14.6368, 20.4406) -> (14.6368, 21.0756)
  line L573 (49.45, 0.1) -> (49.45, -1)
  line L574 (46.72, -1) -> (46.72, 0)
  line L575 (43.49, 0.1) -> (43.49, 4)
  arc A143 (13.7795, 21.0757) -> (13.4937, 20.7899) centre (13.7795, 20.7899) ccw
  line L576 (13.7477, 34.2519) -> (13.4938, 34.5694)
  line L577 (14.3828, 19.4844) -> (13.7477, 19.4844)
  line L578 (15.5893, 32.639) -> (32.3533, 32.639)
  line L579 (32.3533, 24.6698) -> (15.5893, 24.6698)
  line L580 (15.5893, 18.8278) -> (15.5893, 20.7327)
  arc A144 (48.95, 3) -> (47.95, 3) centre (48.45, 3) ccw
  line L581 (45.49, 0.1) -> (45.49, 4)
  line L582 (14.6368, 32.5755) -> (14.6368, 32.8295)
  arc A145 (15.5893, 20.7328) -> (15.5893, 22.7648) centre (15.5893, 21.7488) ccw
  line L583 (42.76, 0) -> (42.26, 0)
  line L584 (50.68, 0) -> (50.18, 0)
  arc A146 (44.99, 3) -> (43.99, 3) centre (44.49, 3) ccw
  arc A147 (47.95, 2) -> (48.95, 2) centre (48.45, 2) ccw
  line L585 (47.95, 3) -> (47.95, 2)
  line L586 (32.3533, 24.6698) -> (32.3533, 18.8278)
  arc A148 (11.8183, 35.9283) -> (12.0779, 36.1879) centre (11.8183, 36.1879) ccw
  line L587 (14.6368, 19.9924) -> (14.6368, 19.7384)
  line L588 (13.4938, 33.5497) -> (13.4938, 33.8037)
  line L589 (14.6368, 34.2519) -> (14.6368, 34.8869)
  line L590 (15.5893, 18.8278) -> (32.3533, 18.8278)
  line L591 (32.3533, 38.481) -> (32.3533, 32.639)
  line L592 (15.5893, 24.6698) -> (15.5893, 22.7647)
  arc A149 (43.99, 2) -> (44.99, 2) centre (44.49, 2) ccw
  line L593 (13.4938, 18.8912) -> (14.6368, 18.8912)
  line L594 (12.078, 25.4538) -> (12.078, 25.1942)
  line L595 (13.4938, 18.7643) -> (13.4938, 19.0183)
  arc A150 (14.3828, 19.4844) -> (14.6368, 19.7384) centre (14.3828, 19.7384) ccw
  line L596 (11.8183, 35.9283) -> (11.1692, 35.9283)
  line L597 (13.4938, 32.7025) -> (14.6368, 32.7025)
  line L598 (11.4288, 26.2798) -> (11.4288, 26.0202)
  line L599 (14.6368, 18.7643) -> (14.6368, 19.0183)
  line L600 (49.45, 0.1) -> (49.45, 4)
  arc A151 (13.4937, 19.7384) -> (13.7477, 19.4844) centre (13.7477, 19.7384) ccw
  arc A152 (14.0017, 20.9804) -> (13.7795, 21.0756) centre (13.7795, 20.7687) ccw
  line L601 (10.9096, 25.8904) -> (10.9096, 26.2798)
  arc A153 (13.4938, 20.7899) -> (13.7478, 20.4407) centre (13.8609, 20.7899) ccw
  line L602 (48.95, 3) -> (48.95, 2)
  line L603 (14.6368, 33.8037) -> (14.6368, 33.5497)
  arc A154 (13.4937, 33.5497) -> (13.7477, 33.2957) centre (13.7477, 33.5497) ccw
  line L604 (43.0542, 30.3851) -> (43.0542, 30.7097)
  line L605 (49.524, 37.286) -> (49.524, 37.794)
  line L606 (46.476, 32.206) -> (46.984, 32.206)
  line L607 (18.11, 46.6662) -> (18.11, 46.825)
  line L608 (49.016, 35.254) -> (49.016, 34.746)
  line L609 (46.984, 39.826) -> (46.984, 40.334)
  line L610 (46.476, 40.334) -> (46.476, 39.826)
  arc A155 (36.2536, 38.9849) -> (36.351, 39.2121) centre (36.0372, 39.2121) ccw
  line L611 (49.524, 40.334) -> (49.016, 40.334)
  line L612 (49.524, 35.254) -> (49.016, 35.254)
  line L613 (24.9362, 53.81) -> (24.9362, 54.6038)
  line L614 (43.0542, 29.5982) -> (43.0542, 29.4683)
  line L615 (49.016, 37.794) -> (49.016, 37.286)
  line L616 (34.6139, 39.5042) -> (34.9384, 39.5042)
  line L617 (49.524, 34.746) -> (49.524, 35.254)
  line L618 (46.476, 35.254) -> (46.476, 34.746)
  arc A156 (42.405, 30.7746) -> (41.8858, 30.7746) centre (42.1454, 30.7746) ccw
  line L619 (49.524, 32.714) -> (49.016, 32.714)
  line L620 (46.476, 37.794) -> (46.476, 37.286)
  line L621 (46.984, 40.334) -> (46.476, 40.334)
  line L622 (49.016, 39.826) -> (49.524, 39.826)
  line L623 (49.016, 37.286) -> (49.524, 37.286)
  line L624 (49.524, 37.794) -> (49.016, 37.794)
  line L625 (46.984, 37.794) -> (46.476, 37.794)
  line L626 (42.4051, 30.7746) -> (42.4051, 30.515)
  arc A157 (43.0542, 30.7097) -> (42.405, 30.7097) centre (42.7296, 30.7097) ccw
  line L627 (46.984, 37.286) -> (46.984, 37.794)
  line L628 (16.84, 48.2537) -> (16.84, 54.6038)
  arc A158 (34.9384, 38.855) -> (34.9384, 39.5042) centre (34.9384, 39.1796) ccw
  line L629 (49.524, 39.826) -> (49.524, 40.334)
  line L630 (46.476, 39.826) -> (46.984, 39.826)
  arc A159 (43.0542, 29.5982) -> (42.7946, 29.8578) centre (42.7946, 29.5982) ccw
  line L631 (37.16, 45.3962) -> (16.84, 45.3962)
  arc A160 (8.9451, 47.6612) -> (8.9451, 48.1804) centre (8.9451, 47.9208) ccw
  line L632 (49.016, 40.334) -> (49.016, 39.826)
  line L633 (35.7018, 38.3358) -> (36.351, 38.3358)
  line L634 (7.4676, 47.0121) -> (7.4676, 48.1805)
  line L635 (41.8858, 30.3851) -> (41.8858, 30.7746)
  arc A161 (36.0589, 39.5042) -> (35.7019, 39.2445) centre (36.0589, 39.1289) ccw
  line L636 (41.8858, 29.8578) -> (42.7946, 29.8578)
  line L637 (46.984, 35.254) -> (46.476, 35.254)
  line L638 (8.5556, 47.0121) -> (8.8801, 47.0121)
  line L639 (46.984, 34.746) -> (46.984, 35.254)
  line L640 (49.016, 32.714) -> (49.016, 32.206)
  line L641 (46.476, 34.746) -> (46.984, 34.746)
  line L642 (46.476, 37.286) -> (46.984, 37.286)
  line L643 (49.016, 32.206) -> (49.524, 32.206)
  line L644 (49.524, 32.206) -> (49.524, 32.714)
  line L645 (49.016, 34.746) -> (49.524, 34.746)
  line L646 (36.3663, 46.19) -> (17.6337, 46.19)
  line L647 (37.16, 48.2537) -> (37.16, 46.825)
  line L648 (24.9362, 53.3338) -> (29.0638, 53.3338)
  line L649 (18.11, 48.2537) -> (18.11, 53.3338)
  line L650 (35.89, 46.6662) -> (18.11, 46.6662)
  line L651 (36.3663, 46.825) -> (37.16, 46.825)
  line L652 (18.11, 53.3338) -> (24.9362, 53.3338)
  line L653 (16.84, 46.825) -> (16.84, 48.2537)
  line L654 (35.89, 46.825) -> (36.3663, 46.825)
  line L655 (16.84, 54.6038) -> (24.9362, 54.6038)
  line L656 (24.9362, 54.6038) -> (29.0638, 54.6038)
  line L657 (18.11, 46.825) -> (17.6337, 46.825)
  line L658 (37.16, 54.6038) -> (37.16, 48.2537)
  line L659 (36.3663, 48.2537) -> (37.16, 48.2537)
  line L660 (35.89, 48.2537) -> (35.89, 46.825)
  line L661 (29.0638, 54.6038) -> (37.16, 54.6038)
  line L662 (17.6337, 48.2537) -> (16.84, 48.2537)
  line L663 (29.0638, 53.3338) -> (35.89, 53.3338)
  line L664 (18.11, 46.825) -> (18.11, 48.2537)
  line L665 (35.89, 48.2537) -> (36.3663, 48.2537)
  line L666 (37.16, 46.825) -> (37.16, 45.3962)
  line L667 (35.89, 46.825) -> (35.89, 46.6662)
  line L668 (29.0638, 53.81) -> (29.0638, 54.6038)
  line L669 (18.11, 48.2537) -> (17.6337, 48.2537)
  line L670 (17.6337, 46.825) -> (16.84, 46.825)
  line L671 (16.84, 45.3962) -> (16.84, 46.825)
  line L672 (24.9362, 53.3338) -> (24.9362, 53.81)
  line L673 (29.0638, 53.3338) -> (29.0638, 53.81)
  line L674 (35.89, 53.3338) -> (35.89, 48.2537)
  line L675 (24.9362, 53.81) -> (17.6337, 53.81)
  line L676 (32.2388, 53.0162) -> (31.9213, 53.0162)
  line L677 (31.7625, 53.0162) -> (32.08, 52.6987)
  line L678 (31.6038, 53.0162) -> (32.08, 52.54)
  line L679 (32.334, 51.524) -> (31.826, 51.524)
  line L680 (31.826, 51.016) -> (32.334, 51.016)
  line L681 (36.3663, 46.19) -> (36.3663, 46.825)
  line L682 (17.6337, 46.825) -> (17.6337, 46.19)
  line L683 (36.3663, 48.2537) -> (36.3663, 53.81)
  line L684 (31.9213, 53.0162) -> (32.08, 52.8575)
  line L685 (18.11, 46.6662) -> (17.6337, 46.19)
  line L686 (5.1626, 34.1945) -> (5.1626, 33.7429)
  line L687 (5.1626, 37.7795) -> (3.537, 37.7795)
  line L688 (7.8613, 14.5225) -> (6.2357, 14.5225)
  line L689 (43.5856, 7.8931) -> (44.1274, 6.2675)
  line L690 (7.8613, 18.7094) -> (7.8613, 18.6191)
  line L691 (43.0437, 6.2675) -> (43.5856, 7.8931)
  line L692 (4.4401, 34.1945) -> (4.6207, 34.1945)
  line L693 (6.2357, 14.5225) -> (6.2357, 14.974)
  arc A162 (3.537, 28.5186) -> (3.7627, 28.2026) centre (3.8711, 28.5186) ccw
  line L694 (4.0788, 34.8873) -> (4.0788, 35.4292)
  arc A163 (7.1389, 14.974) -> (6.2357, 14.974) centre (6.6873, 14.974) ccw
  line L695 (6.7776, 17.3651) -> (7.8613, 17.7264)
  line L696 (7.771, 18.6191) -> (7.771, 18.7094)
  arc A164 (44.6451, 6.4933) -> (45.1869, 6.2675) centre (45.1869, 7.0306) ccw
  arc A165 (7.8613, 20.5921) -> (7.6355, 20.9082) centre (7.5271, 20.5921) ccw
  arc A166 (6.4615, 20.2761) -> (7.0485, 20.1406) centre (7.0485, 21.4802) ccw
  line L697 (3.537, 41.7553) -> (4.8916, 41.7553)
  line L698 (5.1626, 24.9408) -> (5.1626, 25.8439)
  arc A167 (4.4401, 38.2311) -> (3.5369, 38.2311) centre (3.9885, 38.2311) ccw
  line L699 (3.537, 37.7795) -> (3.537, 38.2311)
  arc A168 (4.8013, 39.2556) -> (4.8013, 39.978) centre (4.8013, 39.6168) ccw
  line L700 (4.8916, 33.472) -> (4.4401, 33.472)
  line L701 (4.4401, 39.978) -> (4.8013, 39.978)
  line L702 (4.0788, 40.6708) -> (4.0788, 41.2127)
  line L703 (42.1887, 7.8931) -> (42.5499, 7.8931)
  line L704 (7.5904, 16.0625) -> (7.1388, 16.0625)
  arc A169 (4.3498, 28.0671) -> (4.9368, 28.2026) centre (4.3498, 29.4067) ccw
  line L705 (4.6207, 34.1945) -> (4.6207, 33.472)
  arc A170 (4.8916, 33.472) -> (5.1625, 33.7429) centre (4.8916, 33.7429) ccw
  line L706 (4.5304, 35.9487) -> (4.5304, 37.0324)
  arc A171 (4.4401, 34.1944) -> (4.4401, 33.472) centre (4.4401, 33.8332) ccw
  line L707 (41.8274, 6.6287) -> (41.8274, 7.5318)
  line L708 (7.8613, 18.6191) -> (7.771, 18.6191)
  line L709 (5.1626, 40.6708) -> (4.0788, 40.6708)
  arc A172 (7.5904, 16.0625) -> (7.8613, 16.3334) centre (7.5904, 16.3334) ccw
  line L710 (7.8613, 17.7264) -> (6.7776, 18.0876)
  arc A173 (6.4615, 20.9082) -> (6.2357, 20.5921) centre (6.5699, 20.5921) ccw
  line L711 (7.8613, 16.785) -> (7.8613, 16.3334)
  arc A174 (4.4401, 39.978) -> (4.4401, 39.2556) centre (4.4401, 39.6168) ccw
  line L712 (5.1626, 42.0263) -> (5.1626, 42.1166)
  line L713 (4.8013, 39.2555) -> (4.4401, 39.2555)
  line L714 (43.992, 6.6739) -> (43.1792, 6.6739)
  arc A175 (7.1388, 16.785) -> (7.1388, 16.0626) centre (7.1388, 16.4238) ccw
  arc A176 (7.0485, 21.0436) -> (6.4615, 20.9081) centre (7.0485, 19.704) ccw
  arc A177 (7.6356, 20.276) -> (7.8614, 20.5921) centre (7.5272, 20.5921) ccw
  line L715 (3.537, 30.516) -> (4.711, 30.516)
  line L716 (7.8613, 15.4256) -> (7.1388, 15.0643)
  arc A178 (5.1626, 28.5186) -> (4.9368, 28.8347) centre (4.8284, 28.5186) ccw
  line L717 (7.1388, 14.974) -> (7.1388, 14.5225)
  line L718 (5.1626, 34.8873) -> (4.0788, 34.8873)
  line L719 (4.4401, 38.2311) -> (4.4401, 37.7795)
  arc A179 (45.1869, 6.2675) -> (45.5481, 6.6287) centre (45.1869, 6.6287) ccw
  line L720 (4.0788, 41.2127) -> (4.2594, 41.2127)
  arc A180 (4.8916, 41.7554) -> (5.1625, 42.0263) centre (4.8916, 42.0263) ccw
  line L721 (42.5499, 6.2675) -> (42.1887, 6.2675)
  line L722 (4.0788, 41.5747) -> (4.0788, 42.1166)
  line L723 (4.0788, 35.4292) -> (4.2594, 35.4292)
  line L724 (7.3194, 16.785) -> (7.3194, 16.0625)
  line L725 (7.771, 18.7094) -> (7.8613, 18.7094)
  line L726 (39.2408, 28.6938) -> (39.2408, 28.1745)
  line L727 (12.8588, 43.6088) -> (12.8588, 51.2288)
  line L728 (39.5288, 18.415) -> (39.5288, 26.035)
  line L729 (34.6508, 28.3171) -> (34.6508, 29.4855)
  line L730 (37.6508, 28.1745) -> (37.6508, 29.343)
  arc A181 (41.8275, 6.6287) -> (42.1887, 6.2675) centre (42.1887, 6.6287) ccw
  line L731 (7.1388, 16.785) -> (7.3194, 16.785)
  line L732 (39.0461, 29.343) -> (38.7864, 28.4342)
  line L733 (38.2587, 18.415) -> (38.2587, 17.653)
  line L734 (36.1759, 28.9662) -> (35.9163, 28.9662)
  line L735 (9.5238, 50.3938) -> (9.0046, 50.3938)
  line L736 (35.7864, 28.3171) -> (36.111, 28.3171)
  line L737 (16.0208, 43.2582) -> (16.0208, 43.5828)
  line L738 (9.9133, 51.043) -> (9.7835, 51.043)
  arc A182 (7.6355, 20.9081) -> (7.0485, 21.0436) centre (7.0485, 19.704) ccw
  arc A183 (10.1729, 50.7833) -> (9.9133, 51.0429) centre (9.9133, 50.7833) ccw
  line L739 (16.5401, 44.3938) -> (16.5401, 44.7833)
  line L740 (35.2999, 28.3171) -> (35.0403, 28.8363)
  line L741 (9.0046, 50.3938) -> (9.0046, 51.043)
  line L742 (14.605, 51.2288) -> (14.605, 51.9908)
  line L743 (7.5001, 20.2308) -> (6.5969, 20.9533)
  line L744 (16.8646, 44.3938) -> (16.5401, 44.3938)
  line L745 (37.9754, 28.6938) -> (37.6508, 28.6938)
  line L746 (36.9888, 18.415) -> (39.5288, 18.415)
  arc A184 (6.2357, 20.5921) -> (6.4614, 20.2761) centre (6.5698, 20.5921) ccw
  line L747 (38.2587, 26.035) -> (38.2587, 26.797)
  line L748 (9.0046, 49.2582) -> (9.0046, 49.5828)
  line L749 (37.6508, 29.343) -> (37.9754, 29.343)
  line L750 (9.6537, 49.5828) -> (9.6537, 49.2582)
  line L751 (38.7864, 28.4342) -> (39.4355, 28.4342)
  line L752 (34.1313, 18.415) -> (36.6713, 18.415)
  line L753 (10.3187, 43.6088) -> (12.8588, 43.6088)
  line L754 (16.7997, 45.043) -> (16.8646, 45.043)
  line L755 (36.9888, 26.035) -> (36.9888, 18.415)